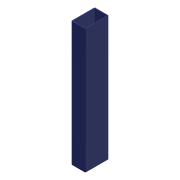
# Autodesk Inventor part: Perfil refuerzo
Saved by Autodesk Inventor 2019 (Build 230136000, 136)
## iProperties
Created: 2020-02-07
Part Number: Perfil refuerzo
Material: Generic
Document SubType Name: Modeling
Designer: Juan Carlos Botero
Density: 1 g/cm^3
Appearance: 48,59,150
Author: Juan Carlos Botero
Autodesk Inventor part; units mm, degrees
ref_plane "YZ Plane" through (0, 0, 0) normal (1, 0, 0) x (0, 1, 0)
ref_plane "XZ Plane" through (0, 0, 0) normal (0, 1, 0) x (-1, 0, 0)
ref_plane "XY Plane" through (0, 0, 0) normal (0, 0, 1) x (1, 0, 0)
sketch "Sketch1" plane through (0, 0, 0) normal (0, 1, 0) x (-1, 0, 0)
  line L0 (30, -50) -> (-30, -50)
  line L1 (-30, -50) -> (-30, 50)
  line L2 (-30, 50) -> (30, 50)
  line L3 (30, 50) -> (30, -50)
  line L4 (30, -50) -> (-30, 50) construction
  line L5 (-30, -50) -> (30, 50) construction
  point P0 (0, 0)
  dimension "d0" = 60
  dimension "d1" = 100
  constraints: 12 end point, 2 midpoint, 2 parallel, 1 horizontal, 1 perpendicular
  measures "d0" distance of L1.end L2.end
  measures "d1" distance of L0.end L1.end
extrude "Extrusion1" add sketch "Sketch1" along normal mid plane 532.5
fillet "Fillet1" radius 3 4 edges at (-30, 0, 50) (30, 0, 50) (30, 0, -50) (-30, 0, -50)
shell "Shell1" thickness 3 removed faces 2 at (10, -266.25, 15.6667) at (10, 266.25, 15.6667)
body "Solid1"
